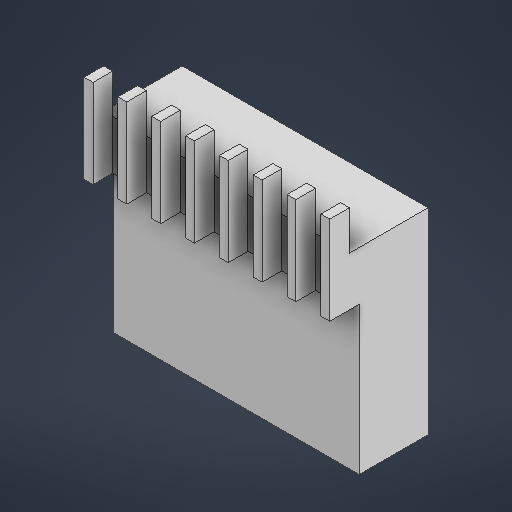
# Autodesk Inventor part: Gyroscope MPU6050
Saved by Autodesk Inventor 2026.2 (Build 302298010, 298A)
## iProperties
Created: 2026-03-17
Part Number: Gyroscope MPU6050
Material: Générique
Document SubType Name: Modeling
Designer: cleml
Density: 1 g/cm^3
Appearance: Par défaut
Author: cleml
Autodesk Inventor part; units mm, degrees
ref_plane "YZ Plane" through (0, 0, 0) normal (1, 0, 0) x (0, 1, 0)
ref_plane "XZ Plane" through (0, 0, 0) normal (0, 1, 0) x (-1, 0, 0)
ref_plane "XY Plane" through (0, 0, 0) normal (0, 0, 1) x (1, 0, 0)
sketch "Esquisse1" plane through (0, 0, 0) normal (0, 0, 1) x (1, 0, 0)
  line L0 (-12.5, -10) -> (12.5, -10)
  line L1 (12.5, -10) -> (12.5, 10)
  line L2 (12.5, 10) -> (-12.5, 10)
  line L3 (-12.5, 10) -> (-12.5, -10)
  line L4 (-12.5, -10) -> (12.5, 10) construction
  line L5 (12.5, -10) -> (-12.5, 10) construction
  point P0 (0, 0)
  dimension "d0" = 25
  dimension "d1" = 20
  constraints: 12 end point, 2 midpoint, 2 parallel, 1 horizontal, 1 perpendicular
  measures "d0" distance of L1.end L2.end
  measures "d1" distance of L0.end L1.end
extrude "Extrusion1" add sketch "Esquisse1" along normal blind 7
sketch "Esquisse2" plane through (0, 0, 7) normal (0, 0, 1) x (1, 0, 0)
  line L0 (12.5, -10) -> (12.5, 10) projected
  line L1 (-12.5, 10) -> (-12.5, -10) projected
  line L2 (12.5, 10) -> (-12.5, 10)
  line L3 (-12.5, 10) -> (-12.5, 5)
  line L4 (-12.5, 5) -> (12.5, 5)
  line L5 (12.5, 5) -> (12.5, 10)
  point P0 (0, 0)
  point P1 (12.5, 5)
  dimension "d4" = 5
  constraints: 8 end point, 2 parallel, 1 horizontal, 1 perpendicular, 1 point on line
  measures "d4" distance between parallel lines of L2 L4
extrude "Extrusion2" add sketch "Esquisse2" along normal blind 3
sketch "Esquisse3" plane through (-12.5, 10, 0) normal (0, 1, 0) x (1, 0, 0)
  line L0 (25, 0) -> (25, -10) projected
  line L1 (25, -10) -> (24.1, -10)
  line L2 (24.1, -10) -> (24.1, -8)
  line L3 (24.1, -8) -> (25, -8)
  line L4 (25, -8) -> (25, -10)
  line L5 (24.1, -10) -> (21.56, -10)
  line L6 (25, -10) -> (0, -10) projected
  line L7 (21.56, -10) -> (16.1469, -10)
  line L8 (21.56, -10) -> (20.66, -10)
  line L9 (20.66, -10) -> (20.66, -8)
  line L10 (20.66, -8) -> (21.56, -8)
  line L11 (21.56, -8) -> (21.56, -10)
  line L12 (20.66, -10) -> (18.12, -10)
  line L13 (18.12, -10) -> (17.22, -10)
  line L14 (17.22, -10) -> (17.22, -8)
  line L15 (17.22, -8) -> (18.12, -8)
  line L16 (18.12, -8) -> (18.12, -10)
  line L17 (17.22, -10) -> (14.68, -10)
  line L18 (14.68, -10) -> (13.78, -10)
  line L19 (13.78, -10) -> (13.78, -8)
  line L20 (13.78, -8) -> (14.68, -8)
  line L21 (14.68, -8) -> (14.68, -10)
  line L22 (13.78, -10) -> (11.24, -10)
  line L23 (11.24, -10) -> (10.34, -10)
  line L24 (10.34, -10) -> (10.34, -8)
  line L25 (10.34, -8) -> (11.24, -8)
  line L26 (11.24, -8) -> (11.24, -10)
  line L27 (10.34, -10) -> (7.8, -10)
  line L28 (7.8, -10) -> (6.9, -10)
  line L29 (6.9, -10) -> (6.9, -8)
  line L30 (6.9, -8) -> (7.8, -8)
  line L31 (7.8, -8) -> (7.8, -10)
  line L32 (6.9, -10) -> (4.36, -10)
  line L33 (4.36, -10) -> (3.46, -10)
  line L34 (3.46, -10) -> (3.46, -8)
  line L35 (3.46, -8) -> (4.36, -8)
  line L36 (4.36, -8) -> (4.36, -10)
  line L37 (3.46, -10) -> (0.92, -10)
  line L38 (0.92, -10) -> (0.02, -10)
  line L39 (0.02, -8) -> (0.92, -8)
  line L40 (0.92, -8) -> (0.92, -10)
  line L41 (0, -10) -> (0, -8)
  line L42 (0, -8) -> (0.02, -8)
  point P0 (12.5, 0)
  point P1 (3.46, -10)
  point P2 (4.36, -10)
  point P3 (6.9, -10)
  point P4 (7.8, -10)
  dimension "d7" = 2.54
  dimension "d11" = 0.9
  dimension "d12" = 2
  dimension "d13" = 2.54
  dimension "d14" = 0.9
  dimension "d15" = 2
  dimension "d16" = 2.54
  dimension "d17" = 0.9
  dimension "d18" = 2
  dimension "d19" = 2.54
  dimension "d20" = 0.9
  dimension "d21" = 2
  dimension "d22" = 2.54
  dimension "d23" = 0.9
  dimension "d24" = 2
  dimension "d25" = 2.54
  dimension "d26" = 0.9
  dimension "d27" = 2
  dimension "d28" = 2.54
  dimension "d29" = 0.9
  dimension "d30" = 2
  dimension "d33" = 2
  constraints: 82 end point, 15 parallel, 10 horizontal, 7 perpendicular, 1 point on line, 1 vertical
  measures "d7" distance of L1.end L5.end
  measures "d11" distance of L2.end L3.end
  measures "d12" distance of L1.end L2.end
  measures "d13" distance of L8.end L12.end
  measures "d14" distance of L9.end L10.end
  measures "d15" distance of L8.end L9.end
  measures "d16" distance of L13.end L17.end
  measures "d17" distance of L14.end L15.end
  measures "d18" distance of L13.end L14.end
  measures "d19" distance of L18.end L22.end
  measures "d20" distance of L19.end L20.end
  measures "d21" distance of L18.end L19.end
  measures "d22" distance of L23.end L27.end
  measures "d23" distance of L24.end L25.end
  measures "d24" distance of L23.end L24.end
  measures "d25" distance of L28.end L32.end
  measures "d26" distance of L29.end L30.end
  measures "d27" distance of L28.end L29.end
  measures "d28" distance of L33.end L37.end
  measures "d29" distance of L34.end L35.end
  measures "d30" distance of L33.end L34.end
  measures "d33" distance of L38.end L39.start
extrude "Extrusion3" add sketch "Esquisse3" along normal blind 4
sketch "Esquisse4" plane through (-12.5, 10, 0) normal (0, 1, 0) x (1, 0, 0)
  line L0 (25, -7) -> (25, -10) projected
  line L1 (25, -10) -> (24.1, -10)
  line L2 (0, -10) -> (25, -10) projected
  line L3 (24.1, -10) -> (21.56, -10)
  line L4 (21.56, -10) -> (21.56, -8)
  line L5 (21.56, -8) -> (24.1, -8)
  line L6 (24.1, -8) -> (24.1, -10)
  line L7 (21.56, -10) -> (20.66, -10)
  line L8 (20.66, -10) -> (18.12, -10)
  line L9 (18.12, -10) -> (18.12, -8)
  line L10 (18.12, -8) -> (20.66, -8)
  line L11 (20.66, -8) -> (20.66, -10)
  line L12 (18.12, -10) -> (17.22, -10)
  line L13 (17.22, -10) -> (14.68, -10)
  line L14 (14.68, -10) -> (14.68, -8)
  line L15 (14.68, -8) -> (17.22, -8)
  line L16 (17.22, -8) -> (17.22, -10)
  line L17 (14.68, -10) -> (13.78, -10)
  line L18 (13.78, -10) -> (11.24, -10)
  line L19 (11.24, -10) -> (11.24, -8)
  line L20 (11.24, -8) -> (13.78, -8)
  line L21 (13.78, -8) -> (13.78, -10)
  line L22 (11.24, -10) -> (10.34, -10)
  line L23 (10.34, -10) -> (7.8, -10)
  line L24 (7.8, -10) -> (7.8, -8)
  line L25 (7.8, -8) -> (10.34, -8)
  line L26 (10.34, -8) -> (10.34, -10)
  line L27 (7.8, -10) -> (6.9, -10)
  line L28 (6.9, -10) -> (4.36, -10)
  line L29 (4.36, -10) -> (4.36, -8)
  line L30 (4.36, -8) -> (6.9, -8)
  line L31 (6.9, -8) -> (6.9, -10)
  line L32 (4.36, -10) -> (3.46, -10)
  line L33 (3.46, -10) -> (0.92, -10)
  line L34 (0.92, -10) -> (0.92, -8)
  line L35 (0.92, -8) -> (3.46, -8)
  line L36 (3.46, -8) -> (3.46, -10)
  point P0 (12.5, 0)
  point P1 (3.46, -10)
  point P2 (4.36, -10)
  point P3 (6.9, -10)
  point P4 (7.8, -10)
  dimension "d36" = 0.9
  dimension "d37" = 2.54
  dimension "d38" = 2
  dimension "d39" = 0.9
  dimension "d40" = 2.54
  dimension "d41" = 2
  dimension "d42" = 0.9
  dimension "d43" = 2.54
  dimension "d44" = 2
  dimension "d45" = 0.9
  dimension "d46" = 2.54
  dimension "d47" = 2
  dimension "d48" = 0.9
  dimension "d49" = 2.54
  dimension "d50" = 2
  dimension "d51" = 0.9
  dimension "d52" = 2.54
  dimension "d53" = 2
  dimension "d54" = 0.9
  dimension "d55" = 2.54
  dimension "d56" = 2
  constraints: 70 end point, 14 parallel, 7 horizontal, 7 perpendicular, 1 point on line
  measures "d36" distance of L0.end L1.end
  measures "d37" distance of L4.end L5.end
  measures "d38" distance of L5.end L1.end
  measures "d39" distance of L7.start L7.end
  measures "d40" distance of L9.end L10.end
  measures "d41" distance of L10.end L7.end
  measures "d42" distance of L12.start L12.end
  measures "d43" distance of L14.end L15.end
  measures "d44" distance of L15.end L12.end
  measures "d45" distance of L17.start L17.end
  measures "d46" distance of L19.end L20.end
  measures "d47" distance of L20.end L17.end
  measures "d48" distance of L22.start L22.end
  measures "d49" distance of L24.end L25.end
  measures "d50" distance of L25.end L22.end
  measures "d51" distance of L27.start L27.end
  measures "d52" distance of L29.end L30.end
  measures "d53" distance of L30.end L27.end
  measures "d54" distance of L32.start L32.end
  measures "d55" distance of L34.end L35.end
  measures "d56" distance of L35.end L32.end
extrude "Extrusion4" cut sketch "Esquisse4" along normal through all both and the other way through all
